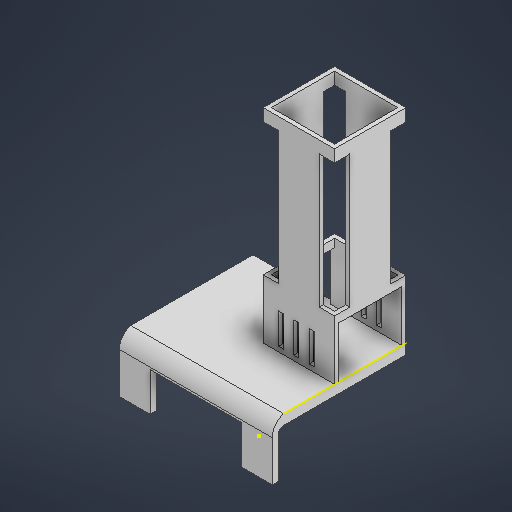
# Autodesk Inventor part: Housing
Saved by Autodesk Inventor 2027 (Build 310192000, 192)
## iProperties
Created: 2026-04-16
Part Number: Housing
Material: Generic
Document SubType Name: Modeling
Designer: ratik
Density: 1 g/cm^3
Appearance: Default
Author: ratik
Autodesk Inventor part; units mm, degrees
ref_plane "YZ Plane" through (0, 0, 0) normal (1, 0, 0) x (0, 1, 0)
ref_plane "XZ Plane" through (0, 0, 0) normal (0, 1, 0) x (-1, 0, 0)
ref_plane "XY Plane" through (0, 0, 0) normal (0, 0, 1) x (1, 0, 0)
sketch "Sketch1" plane through (0, 0, 0) normal (1, 0, 0) x (0, 1, 0)
  line L0 (-8.0203, -13.1567) -> (-48.0203, -13.1567)
  line L1 (-48.0203, -13.1567) -> (-48.0203, -19.1567)
  line L2 (-48.0203, -19.1567) -> (-8.0203, -19.1567)
  line L3 (-3.0203, -24.1567) -> (-3.0203, -144.1567)
  line L4 (-3.0203, -144.1567) -> (6.9797, -144.1567)
  line L5 (6.9797, -144.1567) -> (6.9797, -24.1567)
  arc A0 (6.9797, -24.1567) -> (-8.0203, -13.1567) centre (-7.4798, -28.147) ccw
  arc A1 (-3.0203, -24.1567) -> (-8.0203, -19.1567) centre (-8.0203, -24.1567) ccw
  point P0 (0, 0)
  dimension "d2" = 40
  dimension "d5" = 6
  dimension "d15" = 120
  dimension "d16" = 10
  dimension "d19" = 15
  dimension "d20" = 5
  constraints: 12 end point, 4 point on circle, 2 centre point, 2 parallel, 1 horizontal, 1 perpendicular
  measures "d2" distance of L1.end L2.end
  measures "d5" distance of L0.end L1.end
  measures "d15" distance of L4.end L5.end
  measures "d16" distance of L3.end L4.end
  measures "d19" radius of A0
  measures "d20" radius of A1
extrude "Extrusion1" add sketch "Sketch1" along normal blind 150
sketch "Sketch2" plane through (0, -48.0203, -13.1567) normal (0, 0, 1) x (1, 0, 0)
  line L0 (30, 38) -> (120, 38)
  line L1 (120, 38) -> (120, -15.5969)
  line L2 (120, -15.5969) -> (30, -15.5969)
  line L3 (30, -15.5969) -> (30, 38)
  line L4 (0, 40) -> (150, 40) projected
  line L5 (0, 40) -> (0, 0) projected
  point P0 (0, 48.0203)
  dimension "d10" = 2
  dimension "d11" = 30
  dimension "d12" = 90
  constraints: 8 end point, 2 parallel, 1 horizontal, 1 perpendicular
  measures "d10" distance between parallel lines of L4 L0
  measures "d11" distance between parallel lines of L5 L3
  measures "d12" distance between parallel lines of L1 L3
extrude "Extrusion2" cut sketch "Sketch2" against normal blind 150
sketch "Sketch3" plane through (150, 0, 0) normal (1, 0, 0) x (0, 0, -1)
  line L0 (144.1567, 6.9797) -> (24.1567, 6.9797) projected
  point P0 (0, 0)
sketch "Sketch4" plane through (0, 6.9797, -24.1567) normal (0, 1, 0) x (1, 0, 0)
  line L0 (150, 120) -> (150, 0) projected
  line L1 (150, 120) -> (80, 120)
  line L2 (80, 120) -> (80, 50)
  line L3 (80, 50) -> (150, 50)
  line L4 (150, 50) -> (150, 120)
  point P0 (0, -24.1567)
  dimension "d31" = 70
  dimension "d32" = 70
  constraints: 8 end point, 2 parallel, 1 horizontal, 1 perpendicular
  measures "d31" distance of L1.end L2.end
  measures "d32" distance of L2.end L3.end
extrude "Extrusion3" add sketch "Sketch4" along normal blind 200
sketch "Sketch5" plane through (0, 206.9797, -24.1567) normal (0, 1, 0) x (1, 0, 0)
  line L0 (84, 54) -> (146, 54)
  line L1 (146, 54) -> (146, 116)
  line L2 (146, 116) -> (84, 116)
  line L3 (84, 116) -> (84, 54)
  line L4 (150, 120) -> (80, 120) projected
  line L5 (150, 50) -> (150, 120) projected
  point P0 (0, -24.1567)
  dimension "d35" = 62
  dimension "d36" = 62
  dimension "d37" = 4
  dimension "d38" = 4
  constraints: 8 end point, 2 parallel, 1 horizontal, 1 perpendicular
  measures "d35" distance of L2.end L0.start
  measures "d36" distance of L0.start L0.end
  measures "d37" distance between parallel lines of L4 L2
  measures "d38" distance between parallel lines of L5 L1
extrude "Extrusion4" cut sketch "Sketch5" against normal blind 150
sketch "Sketch6" plane through (150, 0, 0) normal (1, 0, 0) x (0, 0, -1)
  line L0 (78.1567, 6.9797) -> (140.1567, 6.9797)
  line L1 (140.1567, 6.9797) -> (140.1567, 56.9797)
  line L2 (140.1567, 56.9797) -> (78.1567, 56.9797)
  line L3 (78.1567, 56.9797) -> (78.1567, 6.9797)
  line L4 (144.1567, -3.0203) -> (144.1567, 206.9797) projected
  line L5 (74.1567, 6.9797) -> (144.1567, 6.9797) projected
  point P0 (0, 0)
  dimension "d41" = 50
  dimension "d42" = 62
  dimension "d43" = 4
  dimension "d47" = 0
  constraints: 8 end point, 2 parallel, 1 horizontal, 1 perpendicular
  measures "d41" distance of L2.end L0.start
  measures "d42" distance of L1.end L2.end
  measures "d43" distance between parallel lines of L4 L1
  measures "d47" distance between parallel lines of L5 L0
extrude "Extrusion5" cut sketch "Sketch6" against normal blind 150
sketch "Sketch8" plane through (80, 6.9797, -74.1567) normal (0, 0, 1) x (1, 0, 0)
  line L0 (15, 34.7846) -> (20, 34.7846)
  line L1 (20, 34.7846) -> (20, 4.7846)
  line L2 (20, 4.7846) -> (15, 4.7846)
  line L3 (15, 4.7846) -> (15, 34.7846)
  line L4 (30, 34.7846) -> (35, 34.7846)
  line L5 (35, 34.7846) -> (35, 4.7846)
  line L6 (35, 4.7846) -> (30, 4.7846)
  line L7 (30, 4.7846) -> (30, 34.7846)
  line L8 (45, 34.7846) -> (50, 34.7846)
  line L9 (50, 34.7846) -> (50, 4.7846)
  line L10 (50, 4.7846) -> (45, 4.7846)
  line L11 (45, 4.7846) -> (45, 34.7846)
  line L12 (0, 0) -> (0, 200) projected
  point P0 (-80, -6.9797)
  dimension "d48" = 5
  dimension "d49" = 30
  dimension "d50" = 5
  dimension "d51" = 30
  dimension "d52" = 5
  dimension "d53" = 30
  dimension "d54" = 0
  dimension "d55" = 0
  dimension "d56" = 10
  dimension "d57" = 10
  dimension "d58" = 15
  constraints: 24 end point, 6 parallel, 3 horizontal, 3 perpendicular
  measures "d48" distance of L0.start L0.end
  measures "d49" distance of L0.end L1.end
  measures "d50" distance of L4.start L4.end
  measures "d51" distance of L4.end L5.end
  measures "d52" distance of L8.start L8.end
  measures "d53" distance of L8.end L9.end
  measures "d54" distance between parallel lines of L4 L0
  measures "d55" distance between parallel lines of L8 L4
  measures "d56" distance between parallel lines of L5 L11
  measures "d57" distance between parallel lines of L1 L7
  measures "d58" distance between parallel lines of L12 L3
extrude "Extrusion6" cut sketch "Sketch8" against normal through all
sketch "Sketch9" plane through (80, 6.9797, -74.1567) normal (0, 0, 1) x (1, 0, 0)
  line L0 (0, 188.03) -> (15, 188.03)
  line L1 (15, 188.03) -> (15, 58.03)
  line L2 (15, 58.03) -> (0, 58.03)
  line L3 (0, 58.03) -> (0, 188.03)
  line L4 (0, 0) -> (0, 200) projected
  line L5 (55, 188.03) -> (70, 188.03)
  line L6 (70, 188.03) -> (70, 58.03)
  line L7 (70, 58.03) -> (55, 58.03)
  line L8 (55, 58.03) -> (55, 188.03)
  line L9 (70, 0) -> (70, 200) projected
  point P0 (-80, -6.9797)
  dimension "d61" = 0
  dimension "d62" = 15
  dimension "d63" = 130
  dimension "d64" = 15
  dimension "d65" = 130
  dimension "d66" = 0
  dimension "d67" = 0
  constraints: 16 end point, 4 parallel, 2 horizontal, 2 perpendicular
  measures "d61" distance between parallel lines of L4 L3
  measures "d62" distance of L0.start L0.end
  measures "d63" distance of L0.end L1.end
  measures "d64" distance of L5.start L5.end
  measures "d65" distance of L5.end L6.end
  measures "d66" distance between parallel lines of L5 L0
  measures "d67" distance between parallel lines of L9 L6
extrude "Extrusion7" cut sketch "Sketch9" against normal blind 15
sketch "Sketch11" plane through (0, -3.0203, -144.1567) normal (0, 0, -1) x (-1, 0, 0)
  line L0 (-80, 10) -> (-80, 210) projected
  line L1 (-80, 198.03) -> (-95, 198.03)
  line L2 (-95, 198.03) -> (-95, 68.03)
  line L3 (-95, 68.03) -> (-80, 68.03)
  line L4 (-80, 68.03) -> (-80, 198.03)
  line L5 (-135, 197.6999) -> (-150, 197.6999)
  line L6 (-150, 197.6999) -> (-150, 67.6999)
  line L7 (-150, 67.6999) -> (-135, 67.6999)
  line L8 (-135, 67.6999) -> (-135, 197.6999)
  line L9 (-150, 0) -> (-150, 210) projected
  point P0 (0, 3.0203)
  point P1 (-80, 198.03)
  point P2 (-110.828, 197.6999)
  dimension "d71" = 130
  dimension "d72" = 0
  dimension "d73" = 15
  dimension "d74" = 130
  dimension "d75" = 0
  dimension "d76" = 15
  dimension "d77" = 0
  constraints: 16 end point, 4 parallel, 2 horizontal, 2 perpendicular, 1 point on line
  measures "d71" distance of L1.end L2.end
  measures "d72" distance from line of point (-80, 198.03) L1
  measures "d73" distance of L1.start L1.end
  measures "d74" distance of L5.end L6.end
  measures "d75" distance from line of point (-110.828, 197.7) L5
  measures "d76" distance of L5.start L5.end
  measures "d77" distance between parallel lines of L9 L6
extrude "Extrusion8" cut sketch "Sketch11" against normal blind 15
body "Solid1"
